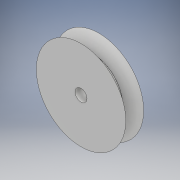
# Autodesk Inventor part: Hand polley
Saved by Autodesk Inventor 2018 (Build 220112000, 112)
## iProperties
Created: 2018-02-14
Part Number: Hand polley
Material: Plastique ABS
Document SubType Name: Modeling
Designer: Thomas
Density: 1.06 g/cm^3
Appearance: Lisse - Blanc
Author: Thomas
Autodesk Inventor part; units mm, degrees
ref_plane "YZ Plane" through (0, 0, 0) normal (1, 0, 0) x (0, 1, 0)
ref_plane "XZ Plane" through (0, 0, 0) normal (0, 1, 0) x (-1, 0, 0)
ref_plane "XY Plane" through (0, 0, 0) normal (0, 0, 1) x (1, 0, 0)
sketch "Esquisse1" plane through (0, 0, 0) normal (0, 0, 1) x (1, 0, 0)
  line L0 (0, 0) -> (0, 2)
  line L1 (0, 2) -> (15, 2)
  line L2 (15, 2) -> (10, 0)
  line L3 (10, 0) -> (0, 0)
  line L4 (0, 0) -> (3.6066, 0) construction
  dimension "d0" = 2
  dimension "d1" = 10
  dimension "d2" = 15
  constraints: 10 end point, 1 horizontal, 1 parallel, 1 perpendicular, 1 vertical
  measures "d0" distance from line of L4 L1.end
  measures "d1" distance of L2.end L0.start
  measures "d2" distance of L0.end L1.end
revolve "Révolution1" add sketch "Esquisse1" angle 360 about axis through (0, 0, 0) along (0, 1, 0)
sketch "Esquisse2" plane through (0, 0, 0) normal (0, -1, 0) x (1, 0, 0)
  circle A0 centre (0, 0) radius 9.9682
  constraints: 1 centre point, 1 coincident
extrude "Extrusion1" add sketch "Esquisse2" along normal blind 2
sketch "Esquisse3" plane through (0, 0, 0) normal (1, 0, 0) x (0, 1, 0)
  line L0 (-2, 9.9682) -> (-2, -9.9682) projected
  line L1 (-2, 0) -> (-2, 9.9682)
  line L2 (-2, 9.9682) -> (-4, 15)
  line L3 (-4, 15) -> (-4, 0)
  line L4 (-4, 0) -> (-2, 0)
  point P0 (0, 0)
  dimension "d6" = 2
  dimension "d7" = 15
  constraints: 8 end point, 1 midpoint, 1 parallel, 1 perpendicular, 1 vertical
  measures "d6" distance of L3.end L1.start
  measures "d7" distance of L2.end L3.end
revolve "Révolution2" add sketch "Esquisse3" angle 360 about axis through (0, -4, 0) along (0, 1, 0)
sketch "Esquisse4" plane through (0, -4, 0) normal (0, -1, 0) x (1, 0, 0)
  circle A0 centre (0, 0) radius 2
  dimension "d9" = 4
  constraints: 1 centre point, 1 coincident
  measures "d9" diameter of A0
extrude "Extrusion2" cut sketch "Esquisse4" against normal blind 6
